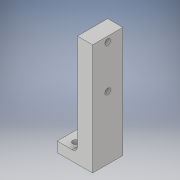
# Autodesk Inventor part: GlyphtMotorBrace
Saved by Autodesk Inventor 2017 (Build 210142000, 142)
## iProperties
Created: 2018-01-10
Part Number: GlyphtMotorBrace
Material: Generic
Document SubType Name: Modeling
Designer: User
Density: 1 g/cm^3
Appearance: Default
Author: User
Autodesk Inventor part; units mm, degrees
ref_plane "YZ Plane" through (0, 0, 0) normal (1, 0, 0) x (0, 1, 0)
ref_plane "XZ Plane" through (0, 0, 0) normal (0, 1, 0) x (-1, 0, 0)
ref_plane "XY Plane" through (0, 0, 0) normal (0, 0, 1) x (1, 0, 0)
sketch "Sketch1" plane through (0, 0, 0) normal (1, 0, 0) x (0, 1, 0)
  line L0 (0, 0) -> (69.85, 0)
  line L1 (69.85, 0) -> (69.85, -19.05)
  line L2 (69.85, -19.05) -> (0, -19.05)
  line L3 (0, -19.05) -> (0, 0)
  dimension "d0" = 19.05
  dimension "d1" = 69.85
  constraints: 8 end point, 2 parallel, 1 horizontal, 1 perpendicular
  measures "d0" distance of L0.end L1.end
  measures "d1" distance of L1.end L2.end
extrude "Extrusion1" add sketch "Sketch1" along normal blind 9.525
sketch "Sketch2" plane through (9.525, 0, 0) normal (1, 0, 0) x (0, 0, -1)
  line L0 (0, 69.85) -> (0, 0) projected
  line L1 (0, 0) -> (19.05, 0) projected
  line L2 (19.05, 0) -> (19.05, 69.85) projected
  line L3 (19.05, 69.85) -> (0, 69.85) projected
  point P0 (9.525, 66.675)
  point P1 (9.525, 39.7256)
  dimension "d4" = 26.9494
  dimension "d5" = 19.05
  dimension "d6" = 69.85
  dimension "d7" = 3.175
  dimension "d8" = 9.525
  dimension "d9" = 9.525
  measures "d4" distance of point (9.525, 39.726) point (9.525, 66.675)
  measures "d5" distance of L2.end L0.start
  measures "d6" distance of L0.start L0.end
  measures "d7" distance from line of L3 point (9.525, 66.675)
  measures "d8" distance from line of L0 point (9.525, 66.675)
  measures "d9" distance from line of L0 point (9.525, 39.726)
hole "Hole1" at (9.525, 66.675, -9.525) at (9.525, 39.7256, -9.525) direction (-1, 0, 0) diameter 3.556 depth 25.4 tip angle 118
sketch "Sketch5" plane through (0, 0, 0) normal (-1, 0, 0) x (0, 0, 1)
  circle A0 centre (-9.525, 66.675) radius 1.778 projected
  circle A1 centre (-9.525, 39.7256) radius 1.778 projected
  line L0 (0, 0) -> (0, 69.85) projected
  line L1 (0, 69.85) -> (-19.05, 69.85) projected
  line L2 (-19.05, 69.85) -> (-19.05, 0) projected
  line L3 (-19.05, 0) -> (0, 0) projected
  line L4 (-19.05, 0) -> (-19.05, 69.85) projected
  line L5 (0, 69.85) -> (0, 0) projected
  line L6 (-19.05, 0) -> (0, 0)
  line L7 (0, 0) -> (0, 6.35)
  line L8 (0, 6.35) -> (-19.05, 6.35)
  line L9 (-19.05, 6.35) -> (-19.05, 0)
  dimension "d31" = 6.35
  constraints: 8 end point, 2 parallel, 1 horizontal, 1 perpendicular, 1 point on line
  measures "d31" distance of L7.end L6.end
extrude "Extrusion2" add sketch "Sketch5" along normal blind 12.7 contours L3 L2 L8 L0
sketch "Sketch6" plane through (0, 6.35, 0) normal (0, 1, 0) x (1, 0, 0)
  line L0 (0, 19.05) -> (0, 0) projected
  line L1 (0, 19.05) -> (-12.7, 19.05) projected
  line L2 (-12.7, 0) -> (-12.7, 19.05) projected
  line L3 (0, 0) -> (-12.7, 0) projected
  point P0 (0, 0)
  point P1 (-6.35, 13.97)
  point P2 (-6.35, 5.08)
  dimension "d34" = 19.05
  dimension "d35" = 5.08
  dimension "d36" = 5.08
  measures "d34" distance of L2.start L1.end
  measures "d35" distance from line of L1 point (-6.35, 13.97)
  measures "d36" distance from line of L3 point (-6.35, 5.08)
hole "Hole3" at (-6.35, 6.35, -13.97) at (-6.35, 6.35, -5.08) direction (0, -1, 0) diameter 3.556 depth 25.4 tip angle 118
fillet "Fillet1" radius 3.175 1 edges at (0, 6.35, -9.525)
equation "\"d8\" = 0.5 * d5"
equation "\"d9\" = d8"
equation "\"d36\" = d35"
body "Solid1"
